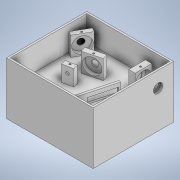
# Autodesk Inventor part: box
Saved by Autodesk Inventor 2022 (Build 260153000, 153)
## iProperties
Created: 2021-07-10
Part Number: box
Material: 常规
Document SubType Name: Modeling
Designer: peter
Density: 1 g/cm^3
Appearance: 默认
Author: peter
Autodesk Inventor part; units mm, degrees
ref_plane "YZ Plane" through (0, 0, 0) normal (1, 0, 0) x (0, 1, 0)
ref_plane "XZ Plane" through (0, 0, 0) normal (0, 1, 0) x (-1, 0, 0)
ref_plane "XY Plane" through (0, 0, 0) normal (0, 0, 1) x (1, 0, 0)
sketch "草图1" plane through (0, 0, 0) normal (0, 1, 0) x (-1, 0, 0)
  line L0 (140.0002, 130) -> (0.0002, 130)
  line L1 (0.0002, 130) -> (0.0002, 0)
  line L2 (0.0002, 0) -> (140.0002, 0)
  line L3 (140.0002, 0) -> (140.0002, 130)
  line L4 (32.8602, 25) -> (32.8602, 12.5)
  line L5 (32.8602, 12.5) -> (32.8602, 37.5)
  line L6 (121.5188, 23.9917) -> (115.2688, 13.1664)
  line L7 (115.2688, 13.1664) -> (127.7688, 34.817)
  line L8 (121.5188, 23.9917) -> (121.0684, 24.2517)
  line L9 (121.0684, 24.2517) -> (115.7522, 15.0437)
  line L10 (115.7522, 15.0437) -> (128.2522, 36.6943)
  line L11 (121.5188, 23.9917) -> (126.7149, 20.9917)
  line L12 (126.7149, 20.9917) -> (120.9441, 10.9963)
  line L13 (120.9441, 10.9963) -> (133.8941, 33.4264)
  line L14 (96.9684, 77.0971) -> (99.5791, 77.6082)
  line L15 (99.5791, 77.6082) -> (87.1157, 75.1682)
  line L16 (87.1157, 75.1682) -> (88.2685, 69.28)
  line L17 (88.2685, 69.28) -> (100.7319, 71.72)
  line L18 (100.7319, 71.72) -> (99.5791, 77.6082)
  line L19 (34.0002, 79.9997) -> (30.2342, 65.9455)
  line L20 (30.2342, 65.9455) -> (37.7662, 94.0539)
  line L21 (33.8602, 38.5) -> (23.5002, 38.5)
  line L22 (23.5002, 38.5) -> (23.5002, 11.5)
  line L23 (23.5002, 11.5) -> (33.8602, 11.5)
  line L24 (33.8602, 11.5) -> (33.8602, 38.5)
  line L25 (135.2601, 33.7924) -> (121.3101, 9.6303)
  line L26 (121.3101, 9.6303) -> (114.7976, 13.3903)
  line L27 (114.7976, 13.3903) -> (128.7476, 37.5524)
  line L28 (128.7476, 37.5524) -> (135.2601, 33.7924)
  line L29 (135.2601, 33.7924) -> (163.1601, 33.7924) construction
  line L30 (95.6553, 78.878) -> (101.1576, 79.9552)
  line L31 (101.1576, 79.9552) -> (84.7687, 76.7467)
  line L32 (84.7687, 76.7467) -> (86.3058, 68.8957)
  line L33 (86.3058, 68.8957) -> (102.6946, 72.1043)
  line L34 (102.6946, 72.1043) -> (101.1576, 79.9552)
  line L35 (34.0002, 79.9997) -> (28.6165, 59.9085)
  line L36 (28.6165, 59.9085) -> (27.9694, 57.4937)
  line L37 (27.9694, 57.4937) -> (44.2758, 118.3468)
  line L38 (44.2758, 118.3468) -> (38.9632, 119.7704)
  line L39 (38.9632, 119.7704) -> (22.6568, 58.9173)
  line L40 (22.6568, 58.9173) -> (27.9694, 57.4937)
  line L41 (44.2758, 118.3468) -> (47.6565, 117.4409)
  line L42 (47.6565, 117.4409) -> (31.3501, 56.5878)
  line L43 (31.3501, 56.5878) -> (27.9694, 57.4937)
  line L44 (84.0002, 47) -> (71.9261, 43.7648)
  line L45 (71.9261, 43.7648) -> (96.0743, 50.2352)
  line L46 (84.0002, 47) -> (83.8656, 47.5023)
  line L47 (83.8656, 47.5023) -> (71.7915, 44.267)
  line L48 (71.7915, 44.267) -> (95.9397, 50.7375)
  line L49 (84.0002, 47) -> (85.5531, 41.2044)
  line L50 (85.5531, 41.2044) -> (73.479, 37.9692)
  line L51 (73.479, 37.9692) -> (97.6272, 44.4397)
  line L52 (88.8643, 48.8417) -> (69.8597, 43.7494)
  line L53 (69.8597, 43.7494) -> (97.8715, 51.2552)
  line L54 (81.0721, 37.9332) -> (62.0675, 32.8409)
  line L55 (62.0675, 32.8409) -> (100.0767, 43.0255)
  line L56 (100.0767, 43.0255) -> (97.8715, 51.2552)
  line L57 (97.8715, 51.2552) -> (69.8597, 43.7494)
  line L58 (69.8597, 43.7494) -> (72.0648, 35.5197)
  line L59 (72.0648, 35.5197) -> (100.0767, 43.0255)
  line L60 (101.1576, 79.9552) -> (102.6946, 72.1043)
  line L61 (102.6946, 72.1043) -> (86.3058, 68.8957)
  line L62 (86.3058, 68.8957) -> (84.7687, 76.7467)
  line L63 (84.7687, 76.7467) -> (101.1576, 79.9552)
  line L64 (101.1576, 79.9552) -> (102.6946, 72.1043)
  line L65 (102.6946, 72.1043) -> (86.3058, 68.8957)
  line L66 (86.3058, 68.8957) -> (84.7687, 76.7467)
  line L67 (84.7687, 76.7467) -> (101.1576, 79.9552)
  line L68 (0.0002, 35) -> (8.0002, 35)
  line L69 (8.0002, 35) -> (8.0002, 15)
  line L70 (8.0002, 15) -> (0.0002, 15)
  line L71 (0.0002, 15) -> (0.0002, 35)
  line L72 (25.0002, 25) -> (0.0002, 25)
  line L73 (8.0002, 35) -> (8.0002, 43)
  line L74 (8.0002, 43) -> (0.0002, 43)
  point P0 (0, 0)
  point P1 (-23.0458, 0.0584)
  point P2 (-23.0458, 0.0584)
  point P3 (-23.0458, 0.0584)
  point P4 (94.5002, 70.5)
  point P5 (94.5002, 70.5)
  point P6 (128.2522, 36.6943)
  point P7 (71.7915, 44.267)
  point P8 (69.8597, 43.7494)
  point P9 (72.0648, 35.5197)
  point P10 (95.9397, 50.7375)
  point P11 (8.0002, 25)
  point P12 (0.0002, 15)
  dimension "d0" = 130
  dimension "d1" = 140
  dimension "d2" = 25
  dimension "d3" = 12.5
  dimension "d4" = 25
  dimension "d5" = 12.5
  dimension "d7" = 0.52
  dimension "d8" = 25
  dimension "d9" = 6
  dimension "d11" = 7.86
  dimension "d13" = 12.7
  dimension "d14" = 6
  dimension "d30" = 14.55
  dimension "d31" = 29.1
  dimension "d32" = 1
  dimension "d33" = 1
  dimension "d34" = 1
  dimension "d35" = 1.5
  dimension "d36" = 120
  dimension "d37" = 0
  dimension "d38" = 1
  dimension "d39" = 1
  dimension "d40" = 1
  dimension "d45" = 0
  dimension "d46" = 2
  dimension "d47" = 2
  dimension "d48" = 2
  dimension "d49" = 70.5
  dimension "d50" = 96.5186
  dimension "d51" = 94.5
  dimension "d52" = 34
  dimension "d53" = 65.9455
  dimension "d68" = 20.8
  dimension "d69" = 2.5
  dimension "d70" = 63
  dimension "d71" = 5.5
  dimension "d72" = 63
  dimension "d73" = 3.5
  dimension "d74" = 84
  dimension "d75" = 47
  dimension "d76" = 12.5
  dimension "d77" = 25
  dimension "d78" = 0.52
  dimension "d79" = 6
  dimension "d84" = 14.5
  dimension "d85" = 14.5
  dimension "d86" = 0
  dimension "d87" = 2
  dimension "d113" = 27.9
  dimension "d163" = 20
  dimension "d165" = 0
  dimension "d166" = 8
  dimension "d179" = 8
  constraints: 150 end point, 26 perpendicular, 17 equal length, 17 point on line, 5 coincident, 4 midpoint, 3 horizontal, 2 vertical
  measures "d0" distance between parallel lines of L2 L0
  measures "d1" distance between parallel lines of L1 L3
  measures "d2" distance from line of L2 point (25, 25)
  measures "d3" distance of L4.start L4.end
  measures "d4" distance of L4.end L5.end
  measures "d5" distance of L6.start L6.end
  measures "d7" distance of L6.start L8.end
  measures "d8" distance of L9.end L10.end
  measures "d9" distance of L6.start L11.end
  measures "d11" distance of L72.start L4.start
  measures "d13" distance of L14.end L15.end
  measures "d14" distance of L15.end L16.end
  measures "d30" distance of L19.start L19.end
  measures "d31" distance of L19.end L20.end
  measures "d32" distance from line of L4.start L24
  measures "d33" distance from line of L21 L5.end
  measures "d34" distance from line of L23 L4.end
  measures "d35" distance from line of L72.start L22
  measures "d36" angle of L25 L29
  measures "d37" distance between parallel lines of L10 L27
  measures "d38" distance between parallel lines of L25 L13
  measures "d39" distance from line of L28 L13.end
  measures "d40" distance from line of L26 L12.end
  measures "d45" distance between parallel lines of L33 L17
  measures "d46" distance between parallel lines of L15 L31
  measures "d47" distance between parallel lines of L34 L18
  measures "d48" distance between parallel lines of L32 L16
  measures "d49" distance from line of L2 point (94.5, 70.5)
  measures "d50" horizontal distance of L72.start L6.start
  measures "d51" distance from line of L1 point (94.5, 70.5)
  measures "d52" distance from line of L1 L19.start
  measures "d53" distance from line of L2 L19.end
  measures "d68" distance of L19.start L35.end
  measures "d69" distance of L35.end L36.end
  measures "d70" distance of L36.end L37.end
  measures "d71" distance of L37.end L38.end
  measures "d72" distance of L38.end L39.end
  measures "d73" distance of L37.end L41.end
  measures "d74" distance from line of L1 L44.start
  measures "d75" distance from line of L2 L44.start
  measures "d76" distance of L44.start L44.end
  measures "d77" distance of L44.end L45.end
  measures "d78" distance of L44.start L46.end
  measures "d79" distance of L44.start L49.end
  measures "d84" distance between parallel lines of L56 L49
  measures "d85" distance between parallel lines of L58 L49
  measures "d86" distance between parallel lines of L57 L48
  measures "d87" distance between parallel lines of L59 L51
  measures "d113" distance between parallel lines of L26 L28
  measures "d163" distance of L68.end L69.end
  measures "d165" distance from line of L72 point (8, 25)
  measures "d166" distance between parallel lines of L71 L69
  measures "d179" distance of L68.end L73.end
extrude "拉伸2" add sketch "草图1" along normal blind 31 contours L10 L27 L28 L25 L26 L9 | L15 L16 L33 L32 L31 L30 L34 L18 L14 | L14 L18 L17 L16 L15 | L24 L23 L22 L21 | L48 L53 L56 L55 L54 L58 L52 L47
extrude "拉伸3" add sketch "草图1" along normal blind 26 contours L20 L37 L41 L42 L43 L36 L35 L19
extrude "拉伸4" add sketch "草图1" against normal blind 5
sketch "草图3" plane through (-23.5002, 31, 38.5) normal (1, 0, 0) x (0, 0, -1)
  circle A0 centre (13.5, -16) radius 12.9
  line L0 (0, -31) -> (27, -31) projected
  line L1 (27, -31) -> (27, 0) projected
  line L2 (38.5, -31) -> (38.5, -36) projected
  dimension "d94" = 25.8
  dimension "d95" = 15
  dimension "d96" = 13.5
  dimension "d208" = 25
  constraints: 1 centre point
  measures "d94" diameter of A0
  measures "d95" distance from line of L0 A0.centre
  measures "d96" distance from line of L1 A0.centre
  measures "d208" distance from line of L2 A0.centre
extrude "拉伸5" cut sketch "草图3" against normal blind 9.86
sketch "草图4" plane through (-33.8602, 31, 11.5) normal (-1, 0, 0) x (0, 0, 1)
  circle A0 centre (13.5, -16) radius 12.9 projected
  circle A1 centre (13.5, -16) radius 7.5
  point P0 (-11.5, -31)
  dimension "d102" = 15
  constraints: 1 centre point, 1 coincident
  measures "d102" diameter of A1
extrude "拉伸6" cut sketch "草图4" against normal blind 1 contours A1
sketch "草图5" plane through (-102.6946, 0, 72.1043) normal (-0.1921274, 0, -0.98137) x (-0.98137, 0, 0.1921274)
  line L0 (-14.8, 21.5) -> (-1.9, 21.5)
  line L1 (-1.9, 21.5) -> (-1.9, 8.4)
  line L2 (-1.9, 8.4) -> (-14.8, 8.4)
  line L3 (-14.8, 8.4) -> (-14.8, 21.5)
  line L4 (0, 0) -> (0, 31) projected
  line L5 (-16.7, 0) -> (-16.7, 31) projected
  line L6 (-16.7, 0) -> (0, 0) projected
  point P0 (-114.6346, 0)
  dimension "d105" = 1.9
  dimension "d106" = 1.9
  dimension "d107" = 13.1
  dimension "d108" = 8.4
  constraints: 8 end point, 2 parallel, 1 horizontal, 1 perpendicular
  measures "d105" distance between parallel lines of L4 L1
  measures "d106" distance between parallel lines of L5 L3
  measures "d107" distance between parallel lines of L0 L2
  measures "d108" distance between parallel lines of L6 L2
extrude "拉伸7" cut sketch "草图5" against normal blind 6.2
sketch "草图6" plane through (-114.7976, 0, 13.3903) normal (0.8660254, 0, 0.5) x (0.5, 0, -0.8660254)
  circle A0 centre (-13.95, 15) radius 12.9
  line L0 (0, 0) -> (0, 31) projected
  line L1 (-27.9, 0) -> (0, 0) projected
  point P0 (68.9951, 0)
  dimension "d111" = 25.8
  dimension "d112" = 13.95
  dimension "d114" = 15
  constraints: 1 centre point
  measures "d111" diameter of A0
  measures "d112" distance from line of L0 A0.centre
  measures "d114" distance from line of L1 A0.centre
extrude "拉伸8" cut sketch "草图6" against normal blind 6.56
sketch "草图7" plane through (-69.8597, 0, 43.7494) normal (0.258819, 0, 0.9659258) x (0.9659258, 0, -0.258819)
  circle A0 centre (-14.5, 15) radius 12.9
  line L0 (-29, 0) -> (0, 0) projected
  line L1 (-29, 0) -> (-29, 31) projected
  point P0 (78.8025, 0)
  dimension "d117" = 25.8
  dimension "d118" = 15
  dimension "d119" = 14.5
  constraints: 1 centre point
  measures "d117" diameter of A0
  measures "d118" distance from line of A0.centre L0
  measures "d119" distance from line of L1 A0.centre
extrude "拉伸9" cut sketch "草图7" against normal blind 6.54
sketch "草图8" plane through (-47.6565, 0, 117.4409) normal (-0.9659225, 0, -0.2588315) x (-0.2588315, 0, 0.9659225)
  line L0 (-18.7, 10.21) -> (-60.5, 10.21)
  line L1 (-60.5, 10.21) -> (-60.5, 19.79)
  line L2 (-60.5, 19.79) -> (-18.7, 19.79)
  line L3 (-18.7, 19.79) -> (-18.7, 10.21)
  line L4 (-63, 0) -> (-63, 26) projected
  line L5 (-63, 0) -> (0, 0) projected
  point P0 (-125.7738, 0)
  dimension "d122" = 41.8
  dimension "d123" = 9.58
  dimension "d124" = 2.5
  dimension "d125" = 10.21
  constraints: 8 end point, 2 parallel, 1 horizontal, 1 perpendicular
  measures "d122" distance of L1.end L2.end
  measures "d123" distance between parallel lines of L2 L0
  measures "d124" distance between parallel lines of L4 L1
  measures "d125" distance between parallel lines of L5 L0
extrude "拉伸10" cut sketch "草图8" against normal up to surface (3.5 mm away)
sketch "草图10" plane through (0, 0, 0) normal (0, 1, 0) x (1, 0, 0)
  line L0 (-140.0002, 0) -> (-140.0002, -130) projected
  line L1 (-0.0002, 0) -> (-140.0002, 0) projected
  line L2 (-140.0002, -130) -> (-0.0002, -130)
  line L3 (-0.0002, -130) -> (-0.0002, 0)
  line L4 (-0.0002, 0) -> (-140.0002, 0)
  line L5 (-140.0002, 0) -> (-140.0002, -130)
  line L6 (-137.0002, -127) -> (-3.0002, -127)
  line L7 (-3.0002, -127) -> (-3.0002, -3)
  line L8 (-3.0002, -3) -> (-137.0002, -3)
  line L9 (-137.0002, -3) -> (-137.0002, -127)
  point P0 (0, 0)
  dimension "d128" = 3
  dimension "d129" = 3
  dimension "d130" = 3
  dimension "d131" = 3
  constraints: 16 end point, 4 parallel, 2 horizontal, 2 perpendicular
  measures "d128" distance between parallel lines of L0 L9
  measures "d129" distance between parallel lines of L2 L6
  measures "d130" distance between parallel lines of L1 L8
  measures "d131" distance between parallel lines of L3 L7
extrude "拉伸11" add sketch "草图10" along normal blind 40
sketch "草图11" plane through (0, -5, 0) normal (0, -1, 0) x (1, 0, 0)
  line L0 (-137.0002, 127) -> (-3.0002, 127) projected
  line L1 (-3.0002, 3) -> (-137.0002, 3) projected
  line L2 (-3.0002, 127) -> (-137.0002, 127)
  line L3 (-137.0002, 127) -> (-137.0002, 3)
  line L4 (-137.0002, 3) -> (-3.0002, 3)
  line L5 (-3.0002, 3) -> (-3.0002, 127)
  line L6 (-0.0002, 0) -> (-0.0002, 130) projected
  line L7 (-0.0002, 130) -> (-140.0002, 130) projected
  line L8 (-140.0002, 0) -> (-0.0002, 0) projected
  line L9 (-0.0002, 130) -> (-140.0002, 130)
  line L10 (-140.0002, 130) -> (-140.0002, 0)
  line L11 (-140.0002, 0) -> (-0.0002, 0)
  line L12 (-0.0002, 0) -> (-0.0002, 130)
  point P0 (0, 0)
  dimension "d134" = 3
  dimension "d135" = 3
  constraints: 16 end point, 4 parallel, 2 horizontal, 2 perpendicular
  measures "d134" distance between parallel lines of L6 L5
  measures "d135" distance between parallel lines of L7 L0
extrude "拉伸12" add sketch "草图11" along normal blind 40
sketch "草图13" plane through (0, 31, 0) normal (0, 1, 0) x (1, 0, 0)
  line L0 (-73.0978, -37.8464) -> (-98.0187, -44.5239) projected
  line L1 (-71.4052, -44.1635) -> (-96.326, -50.8411) projected
  circle A0 centre (-84.7119, -44.3437) radius 1.5
  point P0 (0, 0)
  dimension "d138" = 3
  constraints: 1 centre point, 1 coincident
  measures "d138" diameter of A0
extrude "拉伸13" cut sketch "草图13" against normal blind 2.5
thread "螺纹1" size "M3x0.5" class "6H" standard "ANSI Metric M Profile" full length
sketch "草图16" plane through (0, 31, 0) normal (0, 1, 0) x (1, 0, 0)
  circle A0 centre (-124.6155, -23.8355) radius 1.5
  point P0 (0, 0)
  dimension "d146" = 3
  constraints: 1 centre point
  measures "d146" diameter of A0
extrude "拉伸15" cut sketch "草图16" against normal blind 2.5
thread "螺纹3" size "M3x0.5" class "6H" standard "ANSI Metric M Profile" full length
sketch "草图18" plane through (0, 31, 0) normal (0, 1, 0) x (1, 0, 0)
  line L0 (-102.6946, -72.1043) -> (-101.1576, -79.9552) projected
  line L1 (-101.1576, -79.9552) -> (-102.6946, -72.1043)
  line L2 (-102.6946, -72.1043) -> (-86.3058, -68.8957)
  line L3 (-86.3058, -68.8957) -> (-84.7687, -76.7467)
  line L4 (-84.7687, -76.7467) -> (-101.1576, -79.9552)
  point P0 (0, 0)
  constraints: 8 end point, 3 equal length, 1 perpendicular
extrude "拉伸16" cut sketch "草图18" against normal blind 5
sketch "草图19" plane through (0, 26, 0) normal (0, 1, 0) x (1, 0, 0)
  line L0 (-84.7687, -76.7467) -> (-86.3058, -68.8957) projected
  circle A0 centre (-93.9046, -73.5423) radius 1.5
  point P0 (0, 0)
  point P1 (-100.83, -71.7392)
  point P2 (-99.6388, -77.8237)
  point P3 (-86.9792, -75.3453)
  constraints: 1 centre point
extrude "拉伸17" cut sketch "草图19" against normal blind 2.5
thread "螺纹4" size "M3x0.5" class "6H" standard "ANSI Metric M Profile" full length
sketch "草图20" plane through (0, 0, 0) normal (0, -1, 0) x (1, 0, 0)
  line L0 (-84.7687, 76.7467) -> (-86.3058, 68.8957) projected
  line L1 (-84.7687, 76.7467) -> (-86.3058, 68.8957)
  line L2 (-86.3058, 68.8957) -> (-102.6946, 72.1043)
  line L3 (-102.6946, 72.1043) -> (-101.1576, 79.9552)
  line L4 (-101.1576, 79.9552) -> (-84.7687, 76.7467)
  line L5 (-69.8597, 43.7494) -> (-72.0648, 35.5197) projected
  line L6 (-69.8597, 43.7494) -> (-72.0648, 35.5197)
  line L7 (-72.0648, 35.5197) -> (-100.0767, 43.0255)
  line L8 (-100.0767, 43.0255) -> (-97.8715, 51.2552)
  line L9 (-97.8715, 51.2552) -> (-69.8597, 43.7494)
  line L10 (-135.2601, 33.7924) -> (-128.7476, 37.5524) projected
  line L11 (-135.2601, 33.7924) -> (-121.2359, 9.5018)
  line L12 (-121.2359, 9.5018) -> (-114.7234, 13.2618)
  line L13 (-114.7234, 13.2618) -> (-128.7476, 37.5524)
  line L14 (-128.7476, 37.5524) -> (-135.2601, 33.7924)
  line L15 (-23.5002, 11.5) -> (-33.8602, 11.5) projected
  line L16 (-23.5002, 11.5) -> (-23.5002, 38.5)
  line L17 (-23.5002, 38.5) -> (-33.8602, 38.5)
  line L18 (-33.8602, 38.5) -> (-33.8602, 11.5)
  line L19 (-33.8602, 11.5) -> (-23.5002, 11.5)
  line L20 (-3.0002, 3) -> (-3.0002, 127) projected
  line L21 (-33.8602, 38.5) -> (-23.5002, 38.5) projected
  point P0 (0, 0)
  dimension "d162" = 0
  constraints: 32 end point, 9 parallel, 5 perpendicular, 1 collinear
  measures "d162" distance between parallel lines of L21 L17
extrude "拉伸18" add sketch "草图20" along normal blind 5
extrude "拉伸19" add sketch "草图1" along normal blind 30 contours L74 L73 L68 L1 | L68 L69 L72 L1 | L1 L72 L69 L70
sketch "草图23" plane through (0, 31, 0) normal (0, 1, 0) x (1, 0, 0)
  circle A0 centre (-28.4302, -25) radius 1.5
  point P0 (0, 0)
  point P1 (-33.3602, -12.3)
  dimension "d180" = 3
  constraints: 1 centre point
  measures "d180" diameter of A0
extrude "拉伸22" cut sketch "草图23" against normal blind 2.5
thread "螺纹5" size "M3x0.5" class "6H" standard "ANSI Metric M Profile" full length
sketch "草图28" plane through (-0.0002, 40, 130) normal (1, 0, 0) x (0, 0, -1)
  circle A0 centre (105, -25) radius 7.5 projected
  circle A1 centre (105, -25) radius 7.6
  arc A2 (104.2008, -15.9352) -> (104.2008, -34.0648) centre (105, -25) ccw
  arc A3 (104.2008, -15.9352) -> (105.7992, -15.9352) centre (105, -15.9) ccw
  arc A4 (105.7992, -34.0648) -> (104.2008, -34.0648) centre (105, -34.1) ccw
  arc A5 (105.7992, -34.0648) -> (105.7992, -15.9352) centre (105, -25) ccw
  line L0 (130, -85) -> (130, 0) projected
  point P0 (130, -40)
  dimension "d188" = 15.2
  dimension "d207" = 25
  constraints: 11 point on circle, 5 centre point, 2 coincident
  measures "d188" diameter of A1
  measures "d207" distance from line of L0 A1.centre
extrude "拉伸23" cut sketch "草图28" against normal blind 10.75 contours A0
extrude "拉伸24" cut sketch "草图28" along normal blind 4 from surface at -8 contours A0 | A1 | A3 A5 A4 A2
sketch "草图30" plane through (0, 0, 0) normal (0, -1, 0) x (1, 0, 0)
  line L0 (-44.2758, 118.3468) -> (-27.9694, 57.4937) projected
  line L1 (-27.9694, 57.4937) -> (-31.3501, 56.5878) projected
  line L2 (-27.9694, 57.4937) -> (-31.3501, 56.5878)
  line L3 (-31.3501, 56.5878) -> (-47.6565, 117.4409)
  line L4 (-47.6565, 117.4409) -> (-44.2758, 118.3468)
  line L5 (-44.2758, 118.3468) -> (-27.9694, 57.4937)
  point P0 (0, 0)
  constraints: 8 end point, 3 equal length, 1 perpendicular
extrude "拉伸25" add sketch "草图30" along normal up to surface (5 mm away)
sketch "草图32" plane through (-100.0767, 0, 43.0255) normal (-0.258819, 0, -0.9659258) x (-0.9659258, 0, 0.258819)
  circle A0 centre (-14.5, 15) radius 12.9 projected
  circle A1 centre (-14.5, 15) radius 5
  point P0 (-107.8025, 0)
  dimension "d198" = 10
  constraints: 1 centre point, 1 coincident
  measures "d198" diameter of A1
extrude "拉伸26" cut sketch "草图32" against normal up to surface (1.98 mm away) contours A1
sketch "草图33" plane through (-127.4537, 15, 22.1914) normal (0.8660254, 0, 0.5) x (0.5, 0, -0.8660254)
  circle A0 centre (0, 0) radius 12.9 projected
  circle A1 centre (0, 0) radius 5
  point P0 (82.9451, -15)
  dimension "d201" = 10
  constraints: 1 centre point, 1 coincident
  measures "d201" diameter of A1
extrude "拉伸27" cut sketch "草图33" against normal up to surface (0.96 mm away) contours A1
sketch "草图34" plane through (-101.1576, 0, 79.9552) normal (0.1921274, 0, 0.98137) x (0.98137, 0, -0.1921274)
  circle A0 centre (8.35, 16) radius 2.5
  point P0 (114.6346, 0)
  dimension "d204" = 5
  constraints: 1 centre point
  measures "d204" diameter of A0
extrude "拉伸28" cut sketch "草图34" against normal up to surface (1.8 mm away)
